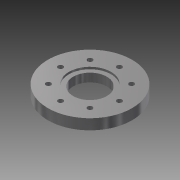
# Autodesk Inventor part: 03
Saved by Autodesk Inventor 2013 (Build 170138000, 138)
## iProperties
Created: 2014-02-07
Material: アルミニウム 6061
Document SubType Name: Modeling
Designer: andou
Density: 2.71 g/cm^3
Mass: 1.57929 g
Surface Area: 8.26239 cm^2
Volume: 0.582765 cm^3
Part Number: 03
Author: andou
Title: Bearing-Holder
Autodesk Inventor part; units mm, degrees
ref_plane "YZ Plane" through (0, 0, 0) normal (1, 0, 0) x (0, 1, 0)
ref_plane "XZ Plane" through (0, 0, 0) normal (0, 1, 0) x (-1, 0, 0)
ref_plane "XY Plane" through (0, 0, 0) normal (0, 0, 1) x (1, 0, 0)
sketch "スケッチ1" plane through (0, 0, 0) normal (0, 0, 1) x (1, 0, 0)
  circle A0 centre (0, 0) radius 10
  dimension "d0" = 20
  constraints: 1 centre point, 1 coincident
  measures "d0" diameter of A0
extrude "押し出し1" add sketch "スケッチ1" along normal blind 2.5
sketch "スケッチ2" plane through (0, 0, 2.5) normal (0, 0, 1) x (1, 0, 0)
  circle A0 centre (0, 0) radius 10 projected
  circle A1 centre (0, 0) radius 4
  dimension "d3" = 8
  constraints: 1 centre point, 1 coincident
  measures "d3" diameter of A1
hole "穴2" at (0, 0, 2.5) direction (0, 0, -1) diameter 8 end through all counterbore diameter 10 counterbore depth 0.5
sketch "スケッチ5" plane through (0, 0, 2.5) normal (0, 0, 1) x (1, 0, 0)
  circle A0 centre (0, 7) radius 0.85
  circle A1 centre (0, 0) radius 5 projected
  dimension "d30" = 1.7
  dimension "d58" = 7
  dimension "d59" = 0
  constraints: 1 centre point
  measures "d30" diameter of A0
  measures "d58" distance of A0.centre A1.centre
  measures "d59" horizontal distance of A1.centre A0.centre
hole "穴4" at (0, 7, 2.5) direction (0, 0, -1) diameter 1.2 end through all
pattern_circular "円形状パターン2" count 8 over 360 about axis through (0, 0, -25.8945) along (0, 0, 1) of "穴4"
